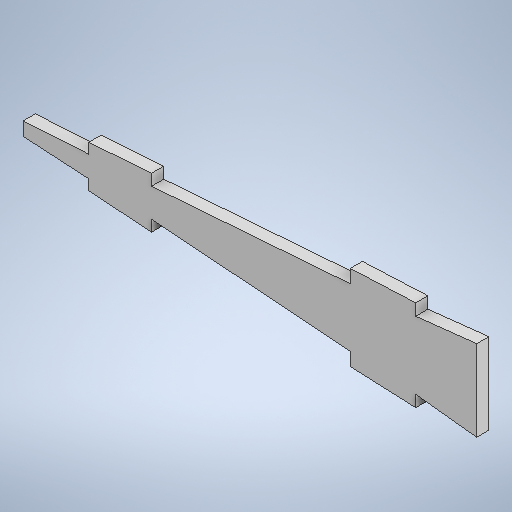
# Autodesk Inventor part: Part3
Saved by Autodesk Inventor 2025.3 (Build 293356000, 356)
## iProperties
Created: 2025-07-04
Part Number: Part3
Material: Generic
Document SubType Name: Modeling
Designer: steve
Density: 1 g/cm^3
Appearance: Default
Author: steve
Autodesk Inventor part; units mm, degrees
ref_plane "YZ Plane" through (0, 0, 0) normal (1, 0, 0) x (0, 1, 0)
ref_plane "XZ Plane" through (0, 0, 0) normal (0, 1, 0) x (-1, 0, 0)
ref_plane "XY Plane" through (0, 0, 0) normal (0, 0, 1) x (1, 0, 0)
sketch "Sketch1" plane through (0, 0, 0) normal (0, 0, 1) x (1, 0, 0)
  line L0 (0, 0) -> (-65, 0)
  line L1 (-65, 0) -> (-65, 3.52)
  line L2 (0, 0) -> (0, 8.315)
  line L3 (0, 0) -> (0, 11.17)
  line L4 (0, 0) -> (15, 0)
  line L5 (15, 0) -> (15, 9.965)
  line L6 (15, 9.965) -> (0, 8.315)
  line L7 (0, 0) -> (-16.11, 0)
  line L8 (-16.11, 0) -> (-16.11, 7.185)
  line L9 (-16.11, 0) -> (-16.11, 10.455)
  line L10 (-65, 0) -> (-65, 6.275)
  line L11 (-65, 0) -> (-80.45, 0)
  line L12 (-80.45, 0) -> (-80.45, 2.625)
  line L13 (-80.45, 0) -> (-80.45, 5.16)
  line L14 (-80.45, 0) -> (-96.59, 0)
  line L15 (-96.59, 0) -> (-96.59, 1.65)
  line L16 (-65, 6.275) -> (-80.45, 5.16)
  line L17 (-96.59, 1.65) -> (-80.45, 2.625)
  line L18 (-65, 3.52) -> (-16.11, 7.185)
  line L19 (0, 11.17) -> (-16.11, 10.455)
  line L20 (-65, 0) -> (-65, -3.52)
  line L21 (0, 0) -> (0, -8.315)
  line L22 (0, 0) -> (0, -11.17)
  line L23 (15, 0) -> (15, -9.965)
  line L24 (15, -9.965) -> (0, -8.315)
  line L25 (-16.11, 0) -> (-16.11, -7.185)
  line L26 (-16.11, 0) -> (-16.11, -10.455)
  line L27 (-65, 0) -> (-65, -6.275)
  line L28 (-80.45, 0) -> (-80.45, -2.625)
  line L29 (-80.45, 0) -> (-80.45, -5.16)
  line L30 (-96.59, 0) -> (-96.59, -1.65)
  line L31 (-65, -6.275) -> (-80.45, -5.16)
  line L32 (-96.59, -1.65) -> (-80.45, -2.625)
  line L33 (-65, -3.52) -> (-16.11, -7.185)
  line L34 (0, -11.17) -> (-16.11, -10.455)
  point P0 (-16.11, -7.185)
  dimension "d0" = 65
  dimension "d1" = 3.52
  dimension "d2" = 8.315
  dimension "d3" = 11.17
  dimension "d4" = 15
  dimension "d6" = 9.965
  dimension "d7" = 16.11
  dimension "d8" = 7.185
  dimension "d9" = 10.455
  dimension "d10" = 6.275
  dimension "d11" = 15.45
  dimension "d12" = 2.625
  dimension "d13" = 5.16
  dimension "d14" = 16.14
  dimension "d15" = 1.65
  constraints: 70 end point, 10 symmetric about line, 6 vertical, 4 horizontal, 4 perpendicular, 1 point on line
  measures "d0" distance of L0.start L0.end
  measures "d1" distance of L0.end L1.end
  measures "d2" distance of L0.start L2.end
  measures "d3" distance of L0.start L3.end
  measures "d4" distance of L0.start L4.end
  measures "d6" distance of L4.end L5.end
  measures "d7" distance of L0.start L7.end
  measures "d8" distance of L7.end L8.end
  measures "d9" distance of L7.end L9.end
  measures "d10" distance of L0.end L10.end
  measures "d11" distance of L0.end L11.end
  measures "d12" distance of L11.end L12.end
  measures "d13" distance of L11.end L13.end
  measures "d14" distance of L11.end L14.end
  measures "d15" distance of L14.end L15.end
extrude "Extrusion1" add sketch "Sketch1" along normal blind 3
body "Solid1"
